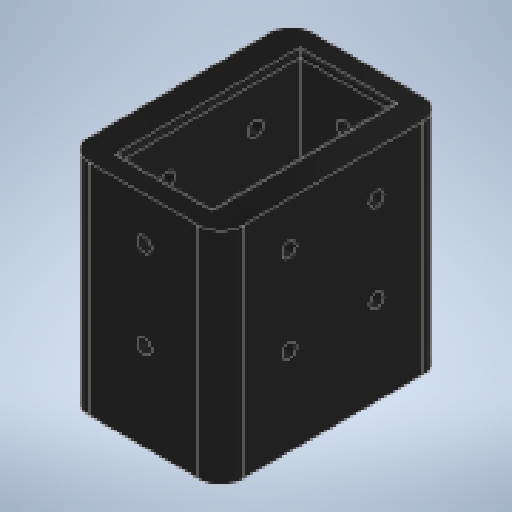
# Autodesk Inventor part: framefixpart2
Saved by Autodesk Inventor 2024.3 (Build 283343010, 343A)
## iProperties
Created: 2025-05-28
Part Number: framefixpart2
Material: 一般
Document SubType Name: Modeling
Designer: kshau
Density: 1 g/cm^3
Appearance: 滑らか - 黒
Mass: 85.4293 g
Surface Area: 201.862 cm^2
Volume: 85.4293 cm^3
Author: kshau
Autodesk Inventor part; units mm, degrees
ref_plane "YZ Plane" through (0, 0, 0) normal (1, 0, 0) x (0, 1, 0)
ref_plane "XZ Plane" through (0, 0, 0) normal (0, 1, 0) x (-1, 0, 0)
ref_plane "XY Plane" through (0, 0, 0) normal (0, 0, 1) x (1, 0, 0)
sketch "スケッチ1" plane through (0, 0, 0) normal (0, 1, 0) x (-1, 0, 0)
  line L0 (0, 0) -> (35, 0)
  line L1 (35, 0) -> (35, -51)
  line L2 (35, -51) -> (0, -51)
  line L3 (0, -51) -> (0, 0)
  dimension "d0" = 35
  dimension "d1" = 51
  constraints: 8 end point, 2 parallel, 1 horizontal, 1 perpendicular
  measures "d0" distance of L0.start L0.end
  measures "d1" distance of L2.end L0.start
extrude "押し出し1" add sketch "スケッチ1" along normal blind 10
sketch "スケッチ2" plane through (0, 10, 0) normal (0, 1, 0) x (1, 0, 0)
  line L0 (-35, 51) -> (-35, 0) projected
  line L1 (-35, 0) -> (0, 0) projected
  line L2 (-17.5, 0) -> (-17.5, 51)
  line L3 (0, 51) -> (-35, 51) projected
  line L4 (-35, 25.5) -> (0, 25.5)
  line L5 (0, 0) -> (0, 51) projected
  line L6 (-17.5, 25.5) -> (-27.6, 25.5)
  line L7 (-27.6, 25.5) -> (-27.6, 45.6)
  line L8 (-27.6, 45.6) -> (-17.5, 45.6)
  line L9 (-17.5, 45.6) -> (-17.5, 25.5)
  line L10 (-27.6, 25.5) -> (-27.6, 5.4)
  line L11 (-27.6, 5.4) -> (-17.5, 5.4)
  line L12 (-7.4, 25.5) -> (-7.4, 45.6)
  line L13 (-7.4, 45.6) -> (-17.5, 45.6)
  line L14 (-7.4, 25.5) -> (-7.4, 5.4)
  line L15 (-7.4, 5.4) -> (-17.5, 5.4)
  dimension "d7" = 20.1
  dimension "d8" = 10.1
  constraints: 24 end point, 5 midpoint, 5 symmetric about line, 2 parallel, 1 horizontal, 1 perpendicular
  measures "d7" distance of L6.end L7.end
  measures "d8" distance of L7.end L8.end
extrude "押し出し2" add sketch "スケッチ2" along normal blind 40 contours L3 L2 L8 L7 L4 L0 | L4 L10 L11 L2 L1 L0 | L3 L5 L4 L12 L13 L2 | L2 L15 L14 L4 L5 L1
fillet "フィレット1" radius 5 4 edges at (0, 25, 0) (0, 25, -51) (-35, 25, -51) (-35, 25, 0)
sketch "スケッチ3" plane through (0, 0, -5) normal (1, 0, 0) x (0, 0, -1)
  line L0 (40.6, 50) -> (0.4, 50) projected
  line L1 (20.5, 50) -> (20.5, 0)
  line L2 (0, 0) -> (41, 0) projected
  line L3 (10.5, 50) -> (10.5, 0)
  line L4 (0, 50) -> (0, 0) projected
  line L5 (0, 10) -> (62, 10)
  line L6 (0.4, 10) -> (40.6, 10) projected
  point P0 (-5, 0)
  point P1 (10.5, 20)
  point P2 (10.5, 40)
  point P3 (30.5, 20)
  point P4 (30.5, 40)
  dimension "d12" = 10
  dimension "d13" = 10
  dimension "d14" = 10
  dimension "d15" = 20
  constraints: 6 end point, 3 point on line, 2 midpoint, 2 symmetric about line, 1 collinear, 1 vertical
  measures "d12" distance between parallel lines of L1 L3
  measures "d13" distance between parallel lines of L2 L5
  measures "d14" distance from line of L5 point (10.5, 20)
  measures "d15" distance of point (10.5, 20) point (10.5, 40)
hole "穴1" at (0, 20, -15.5) at (0, 40, -15.5) at (0, 40, -35.5) at (0, 20, -35.5) direction (-1, 0, 0) diameter 3.3 end through all
sketch "スケッチ4" plane through (-5, 0, -51) normal (0, 0, -1) x (-1, 0, 0)
  line L0 (0, 50) -> (0, 0) projected
  line L1 (0, 10) -> (25, 10)
  line L2 (25, 0) -> (25, 50) projected
  line L3 (0, 0) -> (25, 0) projected
  line L4 (2.4, 50) -> (22.6, 50) projected
  line L5 (12.5, 50) -> (12.5, 10)
  point P0 (-5, 0)
  point P1 (12.5, 20)
  point P2 (12.5, 40)
  dimension "d23" = 10
  dimension "d24" = 10
  dimension "d25" = 20
  constraints: 4 end point, 4 point on line, 2 midpoint, 1 horizontal
  measures "d23" distance between parallel lines of L3 L1
  measures "d24" distance from line of L1 point (12.5, 20)
  measures "d25" distance of point (12.5, 20) point (12.5, 40)
hole "穴2" at (-17.5, 20, -51) at (-17.5, 40, -51) direction (0, 0, 1) diameter 3.3 end through all
sketch "スケッチ5" plane through (0, 0, 0) normal (0, -1, 0) x (1, 0, 0)
  line L0 (-30, 0) -> (-5, 0) projected
  line L1 (-17.5, 0) -> (-17.5, -51)
  line L2 (-15.85, -51) -> (-19.15, -51) projected
  line L3 (0, -5) -> (0, -46) projected
  line L4 (0, -25.5) -> (-35, -25.5)
  line L5 (-35, -46) -> (-35, -5) projected
  point P0 (0, 0)
  point P1 (-17.5, -15.5)
  point P2 (-17.5, -35.5)
  dimension "d33" = 10
  constraints: 4 end point, 4 midpoint, 1 point on line, 1 symmetric about line
  measures "d33" distance from line of L4 point (-17.5, -15.5)
hole "穴3" at (-17.5, 0, -15.5) at (-17.5, 0, -35.5) direction (0, 1, 0) diameter 3.2 end through all
fillet "フィレット2" radius 1 4 edges at (-7.4, 50, -25.5) (-17.5, 50, -5.4) (-27.6, 50, -25.5) (-17.5, 50, -45.6)
sketch "スケッチ6" plane through (0, 0, 0) normal (0, -1, 0) x (1, 0, 0)
  line L0 (-23, -19.5) -> (-12, -19.5)
  line L1 (-12, -19.5) -> (-12, -31.5)
  line L2 (-12, -31.5) -> (-23, -31.5)
  line L3 (-23, -31.5) -> (-23, -19.5)
  circle A0 centre (-17.5, -15.5) radius 1.6 projected
  circle A1 centre (-17.5, -35.5) radius 1.6 projected
  line L4 (0, -5) -> (0, -46) projected
  line L5 (-35, -46) -> (-35, -5) projected
  point P0 (0, 0)
  dimension "d42" = 4
  dimension "d43" = 4
  dimension "d44" = 12
  dimension "d45" = 12
  constraints: 8 end point, 2 parallel, 1 horizontal, 1 perpendicular
  measures "d42" distance from line of A0.centre L0
  measures "d43" distance from line of A1.centre L2
  measures "d44" distance between parallel lines of L4 L1
  measures "d45" distance between parallel lines of L5 L3
extrude "押し出し3" cut sketch "スケッチ6" against normal blind 10 contours L0 L1 L2 L3
